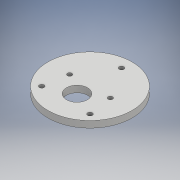
# Autodesk Inventor part: SUPORT STEEP 2
Saved by Autodesk Inventor 2018 (Build 220112000, 112)
## iProperties
Created: 2018-03-05
Part Number: SUPORT STEEP 2
Material: Generic
Document SubType Name: Modeling
Designer: isai
Density: 1 g/cm^3
Appearance: Default
Author: isai
Autodesk Inventor part; units mm, degrees
ref_plane "YZ Plane" through (0, 0, 0) normal (1, 0, 0) x (0, 1, 0)
ref_plane "XZ Plane" through (0, 0, 0) normal (0, 1, 0) x (-1, 0, 0)
ref_plane "XY Plane" through (0, 0, 0) normal (0, 0, 1) x (1, 0, 0)
sketch "Sketch1" plane through (0, 0, 0) normal (0, 0, 1) x (1, 0, 0)
  circle A0 centre (0, 0) radius 32
  circle A1 centre (-15.5, 0) radius 1.7
  circle A2 centre (15.5, 0) radius 1.7
  circle A3 centre (0, -9.9) radius 8
  circle A4 centre (0, 0) radius 18.5
  dimension "d10" = 16
  dimension "d13" = 64
  dimension "d14" = 37
  constraints: 5 centre point, 1 coincident
  measures "d10" diameter of A3
  measures "d13" diameter of A0
  measures "d14" diameter of A4
extrude "Extrusion3" add sketch "Sketch1" along normal blind 5 contours A0 | A4
sketch "Sketch2" plane through (0, 0, 5) normal (0, 0, 1) x (1, 0, 0)
  circle A0 centre (0, -9.9) radius 8 projected
  circle A1 centre (15.5, 0) radius 1.7 projected
  circle A2 centre (-15.5, 0) radius 1.7 projected
  circle A3 centre (0, 0) radius 32 projected
  circle A4 centre (0, 24) radius 1.8
  line L0 (0, 0) -> (-22.6274, -22.6274)
  line L1 (0, 0) -> (-41.0301, 0)
  line L2 (-22.6274, -22.6274) -> (-18.3848, -18.3848)
  circle A5 centre (-18.3848, -18.3848) radius 1.8
  line L3 (0, 0) -> (0, 6.0561)
  circle A6 centre (18.3848, -18.3848) radius 1.8
  dimension "d15" = 3.6
  dimension "d16" = 45
  dimension "d17" = 6
  dimension "d18" = 3.6
  dimension "d21" = 24
  constraints: 8 end point, 3 centre point, 2 coincident, 1 horizontal, 1 point on line, 1 symmetric about line, 1 vertical, 3 other
  measures "d15" diameter of A4
  measures "d16" angle of L0 L1
  measures "d17" distance of L0.end L2.end
  measures "d18" diameter of A5
  measures "d21" distance of A4.centre point (0, 0)
extrude "Extrusion4" cut sketch "Sketch2" against normal up to next contours A5 L0 | L0 A5 | A4 | A6
body "Solid3"
